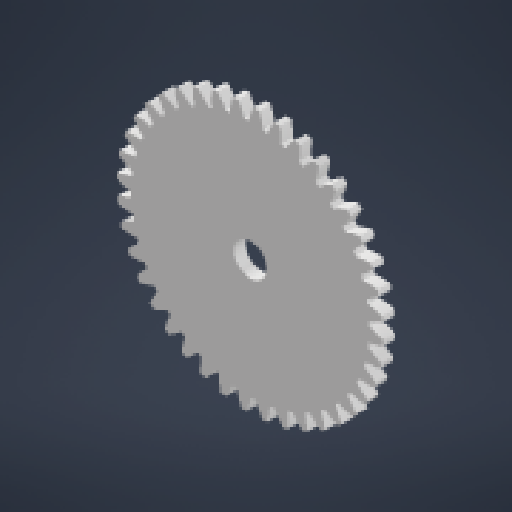
# Autodesk Inventor part: moon_gear_v2
Saved by Autodesk Inventor 2026 (Build 300175050, 175E)
## iProperties
Created: 2026-04-30
Part Number: moon_gear_v2
Material: Generic
Document SubType Name: Modeling
Designer: sniel
Density: 1 g/cm^3
Appearance: Default
Author: sniel
Autodesk Inventor part; units mm, degrees
ref_plane "YZ Plane" through (0, 0, 0) normal (1, 0, 0) x (0, 1, 0)
ref_plane "XZ Plane" through (0, 0, 0) normal (0, 1, 0) x (-1, 0, 0)
ref_plane "XY Plane" through (0, 0, 0) normal (0, 0, 1) x (1, 0, 0)
sketch "Sketch1" plane through (0, 0, 0) normal (0, 0, 1) x (1, 0, 0)
  arc A0 (-17.2509, -28.8749) -> (-16.104, -29.5299) centre (0, 0) ccw
  arc A1 (-16.104, -29.5299) -> (-13.3381, -26.9219) centre (-26.8537, -15.3591) ccw
  arc A2 (-13.3381, -26.9219) -> (-12.2709, -27.4248) centre (0, 0) ccw
  arc A3 (-12.2709, -27.4248) -> (-12.5215, -31.218) centre (5.2503, -30.487) ccw
  arc A4 (-12.5215, -31.218) -> (-11.2862, -31.6855) centre (0, 0) ccw
  arc A5 (-11.2862, -31.6855) -> (-8.9624, -28.6769) centre (-24.1204, -19.3708) ccw
  arc A6 (-8.9624, -28.6769) -> (-7.8296, -29.0067) centre (0, 0) ccw
  arc A7 (-7.8296, -29.0067) -> (-7.4837, -32.7925) centre (9.9549, -29.2904) ccw
  arc A8 (-7.4837, -32.7925) -> (-6.1905, -33.061) centre (0, 0) ccw
  arc A9 (-6.1905, -33.061) -> (-4.366, -29.7259) centre (-20.7932, -22.9056) ccw
  arc A10 (-4.366, -29.7259) -> (-3.1956, -29.8744) centre (0, 0) ccw
  arc A11 (-3.1956, -29.8744) -> (-2.2617, -33.5594) centre (14.4143, -27.3725) ccw
  arc A12 (-2.2617, -33.5594) -> (-0.9424, -33.6224) centre (0, 0) ccw
  arc A13 (-0.9424, -33.6224) -> (0.3379, -30.0429) centre (-16.954, -25.8764) ccw
  arc A14 (0.3379, -30.0429) -> (1.5171, -30.0065) centre (0, 0) ccw
  arc A15 (1.5171, -30.0065) -> (3.016, -33.5001) centre (18.5188, -24.7806) ccw
  arc A16 (3.016, -33.5001) -> (4.3289, -33.3558) centre (0, 0) ccw
  arc A17 (4.3289, -33.3558) -> (5.0335, -29.6202) centre (-12.6973, -28.21) ccw
  arc A18 (5.0335, -29.6202) -> (6.1925, -29.3997) centre (0, 0) ccw
  arc A19 (6.1925, -29.3997) -> (8.2194, -32.6158) centre (22.1674, -21.5785) ccw
  arc A20 (8.2194, -32.6158) -> (9.4936, -32.268) centre (0, 0) ccw
  arc A21 (9.4936, -32.268) -> (9.6052, -28.4681) centre (-8.1279, -29.849) ccw
  arc A22 (9.6052, -28.4681) -> (10.7154, -28.0691) centre (0, 0) ccw
  arc A23 (10.7154, -28.0691) -> (13.2205, -30.9285) centre (25.2701, -17.8451) ccw
  arc A24 (13.2205, -30.9285) -> (14.4245, -30.3856) centre (0, 0) ccw
  arc A25 (14.4245, -30.3856) -> (13.9403, -26.615) centre (-3.3584, -30.753) ccw
  arc A26 (13.9403, -26.615) -> (14.9744, -26.0472) centre (0, 0) ccw
  arc A27 (14.9744, -26.0472) -> (17.896, -28.4796) centre (27.7506, -13.6723) ccw
  arc A28 (17.896, -28.4796) -> (19.0003, -27.755) centre (0, 0) ccw
  arc A29 (19.0003, -27.755) -> (17.9322, -24.1066) centre (1.4937, -30.8997) ccw
  arc A30 (17.9322, -24.1066) -> (18.8648, -23.384) centre (0, 0) ccw
  arc A31 (18.8648, -23.384) -> (22.1308, -25.3294) centre (29.5477, -9.1628) ccw
  arc A32 (22.1308, -25.3294) -> (23.1082, -24.441) centre (0, 0) ccw
  arc A33 (23.1082, -24.441) -> (21.4825, -21.0046) centre (6.3091, -30.2856) ccw
  arc A34 (21.4825, -21.0046) -> (22.2906, -20.145) centre (0, 0) ccw
  arc A35 (22.2906, -20.145) -> (25.8208, -21.5555) centre (30.6173, -4.4277) ccw
  arc A36 (25.8208, -21.5555) -> (26.6471, -20.5252) centre (0, 0) ccw
  arc A37 (26.6471, -20.5252) -> (24.5039, -17.3854) centre (10.9692, -28.9258) ccw
  arc A38 (24.5039, -17.3854) -> (25.1675, -16.41) centre (0, 0) ccw
  arc A39 (25.1675, -16.41) -> (28.8749, -17.2509) centre (30.933, 0.4164) ccw
  arc A40 (28.8749, -17.2509) -> (29.5299, -16.104) centre (0, 0) ccw
  arc A41 (29.5299, -16.104) -> (26.9219, -13.3381) centre (15.3591, -26.8537) ccw
  arc A42 (26.9219, -13.3381) -> (27.4248, -12.2709) centre (0, 0) ccw
  arc A43 (27.4248, -12.2709) -> (31.218, -12.5215) centre (30.487, 5.2503) ccw
  arc A44 (31.218, -12.5215) -> (31.6855, -11.2862) centre (0, 0) ccw
  arc A45 (31.6855, -11.2862) -> (28.6769, -8.9624) centre (19.3708, -24.1204) ccw
  arc A46 (28.6769, -8.9624) -> (29.0067, -7.8296) centre (0, 0) ccw
  arc A47 (29.0067, -7.8296) -> (32.7925, -7.4837) centre (29.2904, 9.9549) ccw
  arc A48 (32.7925, -7.4837) -> (33.061, -6.1905) centre (0, 0) ccw
  arc A49 (33.061, -6.1905) -> (29.7259, -4.366) centre (22.9056, -20.7932) ccw
  arc A50 (29.7259, -4.366) -> (29.8744, -3.1956) centre (0, 0) ccw
  arc A51 (29.8744, -3.1956) -> (33.5594, -2.2617) centre (27.3725, 14.4143) ccw
  arc A52 (33.5594, -2.2617) -> (33.6224, -0.9424) centre (0, 0) ccw
  arc A53 (33.6224, -0.9424) -> (30.0429, 0.3379) centre (25.8764, -16.954) ccw
  arc A54 (30.0429, 0.3379) -> (30.0065, 1.5171) centre (0, 0) ccw
  arc A55 (30.0065, 1.5171) -> (33.5001, 3.016) centre (24.7806, 18.5188) ccw
  arc A56 (33.5001, 3.016) -> (33.3558, 4.3289) centre (0, 0) ccw
  arc A57 (33.3558, 4.3289) -> (29.6202, 5.0335) centre (28.21, -12.6973) ccw
  arc A58 (29.6202, 5.0335) -> (29.3997, 6.1925) centre (0, 0) ccw
  arc A59 (29.3997, 6.1925) -> (32.6158, 8.2194) centre (21.5785, 22.1674) ccw
  arc A60 (32.6158, 8.2194) -> (32.268, 9.4936) centre (0, 0) ccw
  arc A61 (32.268, 9.4936) -> (28.4681, 9.6052) centre (29.849, -8.1279) ccw
  arc A62 (28.4681, 9.6052) -> (28.0691, 10.7154) centre (0, 0) ccw
  arc A63 (28.0691, 10.7154) -> (30.9285, 13.2205) centre (17.8451, 25.2701) ccw
  arc A64 (30.9285, 13.2205) -> (30.3856, 14.4245) centre (0, 0) ccw
  arc A65 (30.3856, 14.4245) -> (26.615, 13.9403) centre (30.753, -3.3584) ccw
  arc A66 (26.615, 13.9403) -> (26.0472, 14.9744) centre (0, 0) ccw
  arc A67 (26.0472, 14.9744) -> (28.4796, 17.896) centre (13.6723, 27.7506) ccw
  arc A68 (28.4796, 17.896) -> (27.755, 19.0003) centre (0, 0) ccw
  arc A69 (27.755, 19.0003) -> (24.1066, 17.9322) centre (30.8997, 1.4937) ccw
  arc A70 (24.1066, 17.9322) -> (23.384, 18.8648) centre (0, 0) ccw
  arc A71 (23.384, 18.8648) -> (25.3294, 22.1308) centre (9.1628, 29.5477) ccw
  arc A72 (25.3294, 22.1308) -> (24.441, 23.1082) centre (0, 0) ccw
  arc A73 (24.441, 23.1082) -> (21.0046, 21.4825) centre (30.2856, 6.3091) ccw
  arc A74 (21.0046, 21.4825) -> (20.145, 22.2906) centre (0, 0) ccw
  arc A75 (20.145, 22.2906) -> (21.5555, 25.8208) centre (4.4277, 30.6173) ccw
  arc A76 (21.5555, 25.8208) -> (20.5252, 26.6471) centre (0, 0) ccw
  arc A77 (20.5252, 26.6471) -> (17.3854, 24.5039) centre (28.9258, 10.9692) ccw
  arc A78 (17.3854, 24.5039) -> (16.41, 25.1675) centre (0, 0) ccw
  arc A79 (16.41, 25.1675) -> (17.2509, 28.8749) centre (-0.4164, 30.933) ccw
  arc A80 (17.2509, 28.8749) -> (16.104, 29.5299) centre (0, 0) ccw
  arc A81 (16.104, 29.5299) -> (13.3381, 26.9219) centre (26.8537, 15.3591) ccw
  arc A82 (13.3381, 26.9219) -> (12.2709, 27.4248) centre (0, 0) ccw
  arc A83 (12.2709, 27.4248) -> (12.5215, 31.218) centre (-5.2503, 30.487) ccw
  arc A84 (12.5215, 31.218) -> (11.2862, 31.6855) centre (0, 0) ccw
  arc A85 (11.2862, 31.6855) -> (8.9624, 28.6769) centre (24.1204, 19.3708) ccw
  arc A86 (8.9624, 28.6769) -> (7.8296, 29.0067) centre (0, 0) ccw
  arc A87 (7.8296, 29.0067) -> (7.4837, 32.7925) centre (-9.9549, 29.2904) ccw
  arc A88 (7.4837, 32.7925) -> (6.1905, 33.061) centre (0, 0) ccw
  arc A89 (6.1905, 33.061) -> (4.366, 29.7259) centre (20.7932, 22.9056) ccw
  arc A90 (4.366, 29.7259) -> (3.1956, 29.8744) centre (0, 0) ccw
  arc A91 (3.1956, 29.8744) -> (2.2617, 33.5594) centre (-14.4143, 27.3725) ccw
  arc A92 (2.2617, 33.5594) -> (0.9424, 33.6224) centre (0, 0) ccw
  arc A93 (0.9424, 33.6224) -> (-0.3379, 30.0429) centre (16.954, 25.8764) ccw
  arc A94 (-0.3379, 30.0429) -> (-1.5171, 30.0065) centre (0, 0) ccw
  arc A95 (-1.5171, 30.0065) -> (-3.016, 33.5001) centre (-18.5188, 24.7806) ccw
  arc A96 (-3.016, 33.5001) -> (-4.3289, 33.3558) centre (0, 0) ccw
  arc A97 (-4.3289, 33.3558) -> (-5.0335, 29.6202) centre (12.6973, 28.21) ccw
  arc A98 (-5.0335, 29.6202) -> (-6.1925, 29.3997) centre (0, 0) ccw
  arc A99 (-6.1925, 29.3997) -> (-8.2194, 32.6158) centre (-22.1674, 21.5785) ccw
  arc A100 (-8.2194, 32.6158) -> (-9.4936, 32.268) centre (0, 0) ccw
  arc A101 (-9.4936, 32.268) -> (-9.6052, 28.4681) centre (8.1279, 29.849) ccw
  arc A102 (-9.6052, 28.4681) -> (-10.7154, 28.0691) centre (0, 0) ccw
  arc A103 (-10.7154, 28.0691) -> (-13.2205, 30.9285) centre (-25.2701, 17.8451) ccw
  arc A104 (-13.2205, 30.9285) -> (-14.4245, 30.3856) centre (0, 0) ccw
  arc A105 (-14.4245, 30.3856) -> (-13.9403, 26.615) centre (3.3584, 30.753) ccw
  arc A106 (-13.9403, 26.615) -> (-14.9744, 26.0472) centre (0, 0) ccw
  arc A107 (-14.9744, 26.0472) -> (-17.896, 28.4796) centre (-27.7506, 13.6723) ccw
  arc A108 (-17.896, 28.4796) -> (-19.0003, 27.755) centre (0, 0) ccw
  arc A109 (-19.0003, 27.755) -> (-17.9322, 24.1066) centre (-1.4937, 30.8997) ccw
  arc A110 (-17.9322, 24.1066) -> (-18.8648, 23.384) centre (0, 0) ccw
  arc A111 (-18.8648, 23.384) -> (-22.1308, 25.3294) centre (-29.5477, 9.1628) ccw
  arc A112 (-22.1308, 25.3294) -> (-23.1082, 24.441) centre (0, 0) ccw
  arc A113 (-23.1082, 24.441) -> (-21.4825, 21.0046) centre (-6.3091, 30.2856) ccw
  arc A114 (-21.4825, 21.0046) -> (-22.2906, 20.145) centre (0, 0) ccw
  arc A115 (-22.2906, 20.145) -> (-25.8208, 21.5555) centre (-30.6173, 4.4277) ccw
  arc A116 (-25.8208, 21.5555) -> (-26.6471, 20.5252) centre (0, 0) ccw
  arc A117 (-26.6471, 20.5252) -> (-24.5039, 17.3854) centre (-10.9692, 28.9258) ccw
  arc A118 (-24.5039, 17.3854) -> (-25.1675, 16.41) centre (0, 0) ccw
  arc A119 (-25.1675, 16.41) -> (-28.8749, 17.2509) centre (-30.933, -0.4164) ccw
  arc A120 (-28.8749, 17.2509) -> (-29.5299, 16.104) centre (0, 0) ccw
  arc A121 (-29.5299, 16.104) -> (-26.9219, 13.3381) centre (-15.3591, 26.8537) ccw
  arc A122 (-26.9219, 13.3381) -> (-27.4248, 12.2709) centre (0, 0) ccw
  arc A123 (-27.4248, 12.2709) -> (-31.218, 12.5215) centre (-30.487, -5.2503) ccw
  arc A124 (-31.218, 12.5215) -> (-31.6855, 11.2862) centre (0, 0) ccw
  arc A125 (-31.6855, 11.2862) -> (-28.6769, 8.9624) centre (-19.3708, 24.1204) ccw
  arc A126 (-28.6769, 8.9624) -> (-29.0067, 7.8296) centre (0, 0) ccw
  arc A127 (-29.0067, 7.8296) -> (-32.7925, 7.4837) centre (-29.2904, -9.9549) ccw
  arc A128 (-32.7925, 7.4837) -> (-33.061, 6.1905) centre (0, 0) ccw
  arc A129 (-33.061, 6.1905) -> (-29.7259, 4.366) centre (-22.9056, 20.7932) ccw
  arc A130 (-29.7259, 4.366) -> (-29.8744, 3.1956) centre (0, 0) ccw
  arc A131 (-29.8744, 3.1956) -> (-33.5594, 2.2617) centre (-27.3725, -14.4143) ccw
  arc A132 (-33.5594, 2.2617) -> (-33.6224, 0.9424) centre (0, 0) ccw
  arc A133 (-33.6224, 0.9424) -> (-30.0429, -0.3379) centre (-25.8764, 16.954) ccw
  arc A134 (-30.0429, -0.3379) -> (-30.0065, -1.5171) centre (0, 0) ccw
  arc A135 (-30.0065, -1.5171) -> (-33.5001, -3.016) centre (-24.7806, -18.5188) ccw
  arc A136 (-33.5001, -3.016) -> (-33.3558, -4.3289) centre (0, 0) ccw
  arc A137 (-33.3558, -4.3289) -> (-29.6202, -5.0335) centre (-28.21, 12.6973) ccw
  arc A138 (-29.6202, -5.0335) -> (-29.3997, -6.1925) centre (0, 0) ccw
  arc A139 (-29.3997, -6.1925) -> (-32.6158, -8.2194) centre (-21.5785, -22.1674) ccw
  arc A140 (-32.6158, -8.2194) -> (-32.268, -9.4936) centre (0, 0) ccw
  arc A141 (-32.268, -9.4936) -> (-28.4681, -9.6052) centre (-29.849, 8.1279) ccw
  arc A142 (-28.4681, -9.6052) -> (-28.0691, -10.7154) centre (0, 0) ccw
  arc A143 (-28.0691, -10.7154) -> (-30.9285, -13.2205) centre (-17.8451, -25.2701) ccw
  arc A144 (-30.9285, -13.2205) -> (-30.3856, -14.4245) centre (0, 0) ccw
  arc A145 (-30.3856, -14.4245) -> (-26.615, -13.9403) centre (-30.753, 3.3584) ccw
  arc A146 (-26.615, -13.9403) -> (-26.0472, -14.9744) centre (0, 0) ccw
  arc A147 (-26.0472, -14.9744) -> (-28.4796, -17.896) centre (-13.6723, -27.7506) ccw
  arc A148 (-28.4796, -17.896) -> (-27.755, -19.0003) centre (0, 0) ccw
  arc A149 (-27.755, -19.0003) -> (-24.1066, -17.9322) centre (-30.8997, -1.4937) ccw
  arc A150 (-24.1066, -17.9322) -> (-23.384, -18.8648) centre (0, 0) ccw
  arc A151 (-23.384, -18.8648) -> (-25.3294, -22.1308) centre (-9.1628, -29.5477) ccw
  arc A152 (-25.3294, -22.1308) -> (-24.441, -23.1082) centre (0, 0) ccw
  arc A153 (-24.441, -23.1082) -> (-21.0046, -21.4825) centre (-30.2856, -6.3091) ccw
  arc A154 (-21.0046, -21.4825) -> (-20.145, -22.2906) centre (0, 0) ccw
  arc A155 (-20.145, -22.2906) -> (-21.5555, -25.8208) centre (-4.4277, -30.6173) ccw
  arc A156 (-21.5555, -25.8208) -> (-20.5252, -26.6471) centre (0, 0) ccw
  arc A157 (-20.5252, -26.6471) -> (-17.3854, -24.5039) centre (-28.9258, -10.9692) ccw
  arc A158 (-17.3854, -24.5039) -> (-16.41, -25.1675) centre (0, 0) ccw
  arc A159 (-16.41, -25.1675) -> (-17.2509, -28.8749) centre (0.4164, -30.933) ccw
  circle A160 centre (0, 0) radius 4.1
  dimension "d0" = 8.2
  constraints: 320 point on circle, 161 centre point, 1 coincident
  measures "d0" diameter of A160
extrude "Extrusion1" add sketch "Sketch1" along normal blind 4
sketch "Sketch3" plane through (0, 0, 0) normal (0, 0, -1) x (-1, 0, 0)
  circle A0 centre (0, 0) radius 5
  circle A1 centre (0, 0) radius 4.1
  dimension "d8" = 10
  constraints: 2 centre point, 1 coincident
  measures "d8" diameter of A0
extrude "Extrusion3" cut sketch "Sketch3" against normal blind 1
body "Solid1"
